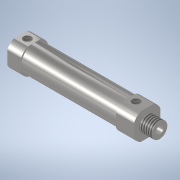
# Autodesk Inventor part: KOGANEI_unkown_35_main
Saved by Autodesk Inventor 2022.3 (Build 263350000, 350)
## iProperties
Created: 2022-04-18
Part Number: KOGANEI_unkown_35_main
Material: ステンレス鋼 440C
Document SubType Name: Modeling
Designer: YusukeKunita
Density: 7.75 g/cm^3
Appearance: 半つや出し
Author: YusukeKunita
Autodesk Inventor part; units mm, degrees
ref_plane "YZ Plane" through (0, 0, 0) normal (1, 0, 0) x (0, 1, 0)
ref_plane "XZ Plane" through (0, 0, 0) normal (0, 1, 0) x (-1, 0, 0)
ref_plane "XY Plane" through (0, 0, 0) normal (0, 0, 1) x (1, 0, 0)
sketch "スケッチ1" plane through (0, 0, 0) normal (0, 1, 0) x (-1, 0, 0)
  circle A0 centre (0, 0) radius 8.5
  dimension "d0" = 17
  constraints: 1 centre point, 1 coincident
  measures "d0" diameter of A0
extrude "押し出し1" add sketch "スケッチ1" along normal blind 61
sketch "スケッチ2" plane through (0, 61, 0) normal (0, 1, 0) x (1, 0, 0)
  circle A0 centre (0, 0) radius 9.5
  line L0 (8.5, -8.5) -> (-8.5, -8.5)
  line L1 (-8.5, -8.5) -> (-8.5, 8.5)
  line L2 (-8.5, 8.5) -> (8.5, 8.5)
  line L3 (8.5, 8.5) -> (8.5, -8.5)
  line L4 (8.5, -8.5) -> (-8.5, 8.5) construction
  line L5 (-8.5, -8.5) -> (8.5, 8.5) construction
  point P0 (8.5, -4.2426)
  point P1 (8.5, 4.2426)
  point P2 (4.2426, 8.5)
  point P3 (-4.2426, 8.5)
  point P4 (-8.5, 4.2426)
  point P5 (-8.5, -4.2426)
  point P6 (-4.2426, -8.5)
  point P7 (4.2426, -8.5)
  dimension "d3" = 19
  dimension "d4" = 17
  dimension "d5" = 17
  constraints: 12 end point, 2 midpoint, 2 parallel, 1 centre point, 1 coincident, 1 horizontal, 1 perpendicular
  measures "d3" diameter of A0
  measures "d4" distance between parallel lines of L2 L0
  measures "d5" distance of L0.start L0.end
extrude "押し出し2" add sketch "スケッチ2" along normal blind 11.6 contours L3 A0 L0 L1 L2
sketch "スケッチ3" plane through (0, 0, 0) normal (0, -1, 0) x (1, 0, 0)
  circle A0 centre (0, 0) radius 9.5
  line L0 (8.5, 8.5) -> (-8.5, 8.5)
  line L1 (-8.5, 8.5) -> (-8.5, -8.5)
  line L2 (-8.5, -8.5) -> (8.5, -8.5)
  line L3 (8.5, -8.5) -> (8.5, 8.5)
  line L4 (8.5, 8.5) -> (-8.5, -8.5) construction
  line L5 (-8.5, 8.5) -> (8.5, -8.5) construction
  point P0 (8.5, -4.2426)
  point P1 (8.5, 4.2426)
  point P2 (4.2426, 8.5)
  point P3 (-4.2426, 8.5)
  point P4 (-8.5, 4.2426)
  point P5 (-8.5, -4.2426)
  point P6 (-4.2426, -8.5)
  point P7 (4.2426, -8.5)
  dimension "d8" = 19
  dimension "d9" = 17
  dimension "d10" = 17
  constraints: 12 end point, 2 midpoint, 2 parallel, 1 centre point, 1 coincident, 1 horizontal, 1 perpendicular
  measures "d8" diameter of A0
  measures "d9" distance of L2.end L0.start
  measures "d10" distance of L1.end L2.end
extrude "押し出し3" add sketch "スケッチ3" along normal blind 9 contours L3 A0 L2 L1 L0
sketch "スケッチ4" plane through (0, 72.6, 0) normal (0, 1, 0) x (1, 0, 0)
  circle A0 centre (0, 0) radius 5
  dimension "d13" = 10
  constraints: 1 centre point, 1 coincident
  measures "d13" diameter of A0
extrude "押し出し4" add sketch "スケッチ4" along normal blind 8
thread "ねじ1" size "M10x1.5" class "6g" standard "ANSI Metric M Profile" full length
sketch "スケッチ5" plane through (-4.2426, 61, 8.5) normal (0, 0, 1) x (1, 0, 0)
  line L0 (0, -61) -> (0, -70) projected
  line L1 (0, 0) -> (0, 11.6) projected
  line L2 (0, 11.6) -> (8.4853, 11.6) projected
  line L3 (0, 0) -> (4.2426, 0) projected
  point P0 (4.2426, -61)
  point P1 (4.2426, 4.5)
  point P2 (4.2426, -65.5)
  point P3 (0, -65.5)
  point P4 (0, 5.8)
  point P5 (4.2426, 11.6)
  dimension "d18" = 4.5
  constraints: 3 midpoint, 2 vertical alignment, 1 horizontal alignment
  measures "d18" distance from line of L3 point (4.243, 4.5)
hole "穴1" at (0, 65.5, 8.5) at (0, -4.5, 8.5) direction (0, 0, -1) diameter 5 depth 10
thread "ねじ2" size "M5x0.8" class "6H" standard "ANSI Metric M Profile" full length
thread "ねじ3" size "M5x0.8" class "6H" standard "ANSI Metric M Profile" full length
sketch "スケッチ6" plane through (0, 80.6, 0) normal (0, 1, 0) x (1, 0, 0)
  circle A0 centre (0, 0) radius 5 projected
  constraints: 1 coincident
hole "穴2" at (0, 80.6, 0) direction (0, -1, 0) diameter 5 depth 80.6
